Autodesk Fusion 360 part; units mm, degrees
note: some values were not read from the file. Set by a fixed rule: which sketch regions a step uses.
(part 2 of 2)
sketch "Sketch46" plane through (0, 0, 3) normal (0, 0, 1) x (-1, 0, 0)
  line L0 (110.0265, 86.5) -> (110.0265, 76.5)
  line L1 (110.0265, 76.5) -> (120.0265, 76.5)
  line L2 (120.0265, 76.5) -> (120.0265, 5)
  line L3 (116.5265, 5) -> (116.5265, 73)
  line L4 (116.5265, 73) -> (106.5265, 73)
  line L5 (106.5265, 73) -> (106.5265, 83)
  line L6 (106.5265, 83) -> (-17.7235, 83)
  line L7 (-21.2235, 86.5) -> (110.0265, 86.5)
  line L8 (-34.7235, -90) -> (123.5265, -90)
  line L9 (123.5265, -90) -> (123.5265, 90)
  line L10 (123.5265, 90) -> (-34.7235, 90)
  line L11 (-34.7235, 90) -> (-34.7235, -90)
  line L12 (12.9015, 40) -> (12.9015, 81)
  line L13 (75.9015, 81) -> (75.9015, 40)
  line L14 (75.9015, 40) -> (12.9015, 40)
  circle A0 centre (59.4015, -45) radius 2.5
  circle A1 centre (59.4015, 15) radius 2.5
  circle A2 centre (59.4015, -15) radius 2.5
  circle A3 centre (78.4015, -45) radius 2.5
  circle A4 centre (78.4015, -15) radius 2.5
  line L15 (-5.7917, -72.9167) -> (-5.7917, -61.9167)
  line L16 (-5.7917, -61.9167) -> (22.9083, -61.9167)
  line L17 (22.9083, -61.9167) -> (22.9083, -72.9167)
  line L18 (22.9083, -72.9167) -> (-5.7917, -72.9167)
  line L19 (-17.7235, -83.5) -> (106.5265, -83.5)
  line L20 (106.5265, -83.5) -> (106.5265, -73)
  line L21 (106.5265, -73) -> (116.5265, -73)
  line L22 (116.5265, -73) -> (116.5265, 0)
  line L23 (116.5265, 0) -> (120.0265, 0)
  line L24 (120.0265, 0) -> (120.0265, -76.5)
  line L25 (120.0265, -76.5) -> (110.0265, -76.5)
  line L26 (110.0265, -76.5) -> (110.0265, -87)
  line L27 (110.0265, -87) -> (-21.2235, -87)
  line L28 (-21.2235, -87) -> (-21.2235, -76.5)
  line L29 (-21.2235, -76.5) -> (-31.2235, -76.5)
  line L30 (-31.2235, -76.5) -> (-31.2235, 0)
  line L31 (-31.2235, 0) -> (-27.7235, 0)
  line L32 (-27.7235, 0) -> (-27.7235, -73)
  line L33 (-27.7235, -73) -> (-17.7235, -73)
  line L34 (-17.7235, -73) -> (-17.7235, -83.5)
  circle A5 centre (116.7765, 83.25) radius 2.5
  line L35 (12.9015, 81) -> (75.9015, 81)
  circle A6 centre (78.4015, 15) radius 2.5
  line L36 (-27.7235, 5) -> (-31.2235, 5)
  line L37 (-31.2235, 5) -> (-31.2235, 76.5)
  line L38 (-31.2235, 76.5) -> (-21.2235, 76.5)
  line L39 (-21.2235, 76.5) -> (-21.2235, 86.5)
  line L40 (-17.7235, 83) -> (-17.7235, 73)
  line L41 (-17.7235, 73) -> (-27.7235, 73)
  line L42 (-27.7235, 73) -> (-27.7235, 5)
  circle A7 centre (-27.9735, 83.25) radius 2.5
  circle A8 centre (10.4015, -15) radius 2.5
  circle A9 centre (10.4015, 15) radius 2.5
  circle A10 centre (29.4015, -45) radius 2.5
  circle A11 centre (29.4015, -15) radius 2.5
  circle A12 centre (29.4015, 15) radius 2.5
  circle A13 centre (10.4015, -45) radius 2.5
  circle A14 centre (-4.7235, 40) radius 3.5
  line L43 (120.0265, 5) -> (116.5265, 5)
  dimension "d201" = 5
  dimension "d350" = 6.75
  measures "d201" diameter of A5
  measures "d350" distance of L10 A5.centre
extrude "Extrude43" cut sketch "Sketch46" against normal blind 3 contours A5 bodies 2
sketch "Sketch47" plane through (0, 0, 3) normal (0, 0, 1) x (-1, 0, 0)
  line L0 (-17.7235, -83.5) -> (106.5265, -83.5)
  line L1 (106.5265, -83.5) -> (106.5265, -73)
  line L2 (106.5265, -73) -> (116.5265, -73)
  line L3 (116.5265, -73) -> (116.5265, 0)
  line L4 (116.5265, 0) -> (120.0265, 0)
  line L5 (120.0265, 0) -> (120.0265, -76.5)
  line L6 (120.0265, -76.5) -> (110.0265, -76.5)
  line L7 (110.0265, -76.5) -> (110.0265, -87)
  line L8 (110.0265, -87) -> (-21.2235, -87)
  line L9 (-21.2235, -87) -> (-21.2235, -76.5)
  line L10 (-21.2235, -76.5) -> (-31.2235, -76.5)
  line L11 (-31.2235, -76.5) -> (-31.2235, 0)
  line L12 (-31.2235, 0) -> (-27.7235, 0)
  line L13 (-27.7235, 0) -> (-27.7235, -73)
  line L14 (-27.7235, -73) -> (-17.7235, -73)
  line L15 (-17.7235, -73) -> (-17.7235, -83.5)
  line L16 (-5.7917, -72.9167) -> (-5.7917, -61.9167)
  line L17 (-5.7917, -61.9167) -> (22.9083, -61.9167)
  line L18 (22.9083, -61.9167) -> (22.9083, -72.9167)
  line L19 (22.9083, -72.9167) -> (-5.7917, -72.9167)
  circle A0 centre (78.4015, -15) radius 2.5
  circle A1 centre (78.4015, -45) radius 2.5
  circle A2 centre (59.4015, -15) radius 2.5
  circle A3 centre (59.4015, 15) radius 2.5
  circle A4 centre (59.4015, -45) radius 2.5
  line L20 (12.9015, 40) -> (12.9015, 81)
  line L21 (12.9015, 81) -> (75.9015, 81)
  line L22 (75.9015, 81) -> (75.9015, 40)
  line L23 (75.9015, 40) -> (12.9015, 40)
  line L24 (-34.7235, -90) -> (123.5265, -90)
  line L25 (123.5265, -90) -> (123.5265, 90)
  line L26 (123.5265, 90) -> (-34.7235, 90)
  line L27 (-34.7235, 90) -> (-34.7235, -90)
  line L28 (110.0265, 86.5) -> (110.0265, 76.5)
  line L29 (110.0265, 76.5) -> (120.0265, 76.5)
  line L30 (120.0265, 76.5) -> (120.0265, 5)
  line L31 (116.5265, 5) -> (116.5265, 73)
  line L32 (116.5265, 73) -> (106.5265, 73)
  line L33 (106.5265, 73) -> (106.5265, 83)
  line L34 (-21.2235, 86.5) -> (110.0265, 86.5)
  line L35 (110.0265, -87) -> (110.0265, -76.5)
  circle A5 centre (116.7765, -83.25) radius 2.5
  line L36 (106.5265, 83) -> (-17.7235, 83)
  circle A6 centre (78.4015, 15) radius 2.5
  line L37 (-17.7235, 83) -> (-17.7235, 73)
  line L38 (-17.7235, 73) -> (-27.7235, 73)
  line L39 (-27.7235, 73) -> (-27.7235, 5)
  line L40 (-27.7235, 5) -> (-31.2235, 5)
  line L41 (-31.2235, 5) -> (-31.2235, 76.5)
  line L42 (-31.2235, 76.5) -> (-21.2235, 76.5)
  line L43 (-21.2235, 76.5) -> (-21.2235, 86.5)
  circle A7 centre (-27.9735, 83.25) radius 2.5
  circle A8 centre (116.7765, 83.25) radius 2.5
  circle A9 centre (10.4015, -45) radius 2.5
  circle A10 centre (29.4015, 15) radius 2.5
  circle A11 centre (29.4015, -15) radius 2.5
  circle A12 centre (29.4015, -45) radius 2.5
  circle A13 centre (10.4015, 15) radius 2.5
  circle A14 centre (10.4015, -15) radius 2.5
  circle A15 centre (-4.7235, 40) radius 3.5
  line L44 (120.0265, 5) -> (116.5265, 5)
  dimension "d204" = 5
  dimension "d351" = 6.75
  constraint coincident L6.end L7.start
  measures "d204" diameter of A5
  measures "d351" distance of L24 A5.centre
extrude "Extrude44" cut sketch "Sketch47" against normal blind 3 contours A5 bodies 2
sketch "Sketch48" plane through (0, 0, 3) normal (0, 0, 1) x (-1, 0, 0)
  line L0 (110.0265, 86.5) -> (110.0265, 76.5)
  line L1 (110.0265, 76.5) -> (120.0265, 76.5)
  line L2 (120.0265, 76.5) -> (120.0265, 5)
  line L3 (116.5265, 5) -> (116.5265, 73)
  line L4 (116.5265, 73) -> (106.5265, 73)
  line L5 (106.5265, 73) -> (106.5265, 83)
  line L6 (106.5265, 83) -> (-17.7235, 83)
  line L7 (-21.2235, 86.5) -> (110.0265, 86.5)
  line L8 (-34.7235, -90) -> (123.5265, -90)
  line L9 (123.5265, -90) -> (123.5265, 90)
  line L10 (123.5265, 90) -> (-34.7235, 90)
  line L11 (-34.7235, 90) -> (-34.7235, -90)
  line L12 (12.9015, 40) -> (12.9015, 81)
  line L13 (75.9015, 81) -> (75.9015, 40)
  line L14 (75.9015, 40) -> (12.9015, 40)
  circle A0 centre (59.4015, -45) radius 2.5
  circle A1 centre (59.4015, 15) radius 2.5
  circle A2 centre (59.4015, -15) radius 2.5
  circle A3 centre (78.4015, -45) radius 2.5
  circle A4 centre (78.4015, -15) radius 2.5
  line L15 (-5.7917, -72.9167) -> (-5.7917, -61.9167)
  line L16 (-5.7917, -61.9167) -> (22.9083, -61.9167)
  line L17 (22.9083, -61.9167) -> (22.9083, -72.9167)
  line L18 (22.9083, -72.9167) -> (-5.7917, -72.9167)
  line L19 (-17.7235, -83.5) -> (106.5265, -83.5)
  line L20 (106.5265, -83.5) -> (106.5265, -73)
  line L21 (106.5265, -73) -> (116.5265, -73)
  line L22 (116.5265, -73) -> (116.5265, 0)
  line L23 (116.5265, 0) -> (120.0265, 0)
  line L24 (120.0265, 0) -> (120.0265, -76.5)
  line L25 (120.0265, -76.5) -> (110.0265, -76.5)
  line L26 (110.0265, -76.5) -> (110.0265, -87)
  line L27 (110.0265, -87) -> (-21.2235, -87)
  line L28 (-21.2235, -87) -> (-21.2235, -76.5)
  line L29 (-21.2235, -76.5) -> (-31.2235, -76.5)
  line L30 (-31.2235, -76.5) -> (-31.2235, 0)
  line L31 (-31.2235, 0) -> (-27.7235, 0)
  line L32 (-27.7235, 0) -> (-27.7235, -73)
  line L33 (-27.7235, -73) -> (-17.7235, -73)
  line L34 (-17.7235, -73) -> (-17.7235, -83.5)
  circle A5 centre (-27.9735, -83.25) radius 2.5
  line L35 (12.9015, 81) -> (75.9015, 81)
  circle A6 centre (78.4015, 15) radius 2.5
  line L36 (-17.7235, 83) -> (-17.7235, 73)
  line L37 (-17.7235, 73) -> (-27.7235, 73)
  line L38 (-27.7235, 73) -> (-27.7235, 5)
  line L39 (-27.7235, 5) -> (-31.2235, 5)
  line L40 (-31.2235, 5) -> (-31.2235, 76.5)
  line L41 (-31.2235, 76.5) -> (-21.2235, 76.5)
  line L42 (-21.2235, 76.5) -> (-21.2235, 86.5)
  circle A7 centre (-27.9735, 83.25) radius 2.5
  circle A8 centre (116.7765, 83.25) radius 2.5
  circle A9 centre (116.7765, -83.25) radius 2.5
  circle A10 centre (10.4015, -15) radius 2.5
  circle A11 centre (10.4015, 15) radius 2.5
  circle A12 centre (29.4015, -45) radius 2.5
  circle A13 centre (29.4015, -15) radius 2.5
  circle A14 centre (29.4015, 15) radius 2.5
  circle A15 centre (10.4015, -45) radius 2.5
  circle A16 centre (-4.7235, 40) radius 3.5
  line L43 (120.0265, 5) -> (116.5265, 5)
  dimension "d207" = 5
  dimension "d352" = 6.75
  measures "d207" diameter of A5
  measures "d352" distance of L8 A5.centre
extrude "Extrude45" cut sketch "Sketch48" against normal blind 3 contours A5 bodies 2
move_body "Move11" bodies 2 to x (1, 0, 0) y (0, 1, 0) z (0, 0, 1) at (274.2168, 184.9353, 0)
sketch "Sketch71" plane through (0, 0, 3) normal (0, 0, 1) x (-1, 0, 0)
  circle A0 centre (-157.4403, -268.1853) radius 2.5
  circle A1 centre (-302.1903, -101.6853) radius 2.5
  line L0 (-291.9403, -268.4353) -> (-167.6903, -268.4353)
  line L1 (-167.6903, -268.4353) -> (-167.6903, -257.9353)
  line L2 (-167.6903, -257.9353) -> (-157.6903, -257.9353)
  line L3 (-157.6903, -257.9353) -> (-157.6903, -184.9353)
  line L4 (-157.6903, -184.9353) -> (-154.1903, -184.9353)
  line L5 (-154.1903, -184.9353) -> (-154.1903, -261.4353)
  line L6 (-154.1903, -261.4353) -> (-164.1903, -261.4353)
  line L7 (-164.1903, -261.4353) -> (-164.1903, -271.9353)
  line L8 (-164.1903, -271.9353) -> (-295.4403, -271.9353)
  line L9 (-295.4403, -271.9353) -> (-295.4403, -261.4353)
  line L10 (-295.4403, -261.4353) -> (-305.4403, -261.4353)
  line L11 (-305.4403, -261.4353) -> (-305.4403, -184.9353)
  line L12 (-305.4403, -184.9353) -> (-301.9403, -184.9353)
  line L13 (-301.9403, -184.9353) -> (-301.9403, -257.9353)
  line L14 (-301.9403, -257.9353) -> (-291.9403, -257.9353)
  line L15 (-291.9403, -257.9353) -> (-291.9403, -268.4353)
  circle A2 centre (-278.9403, -144.9353) radius 3.5
  line L16 (-308.9403, -274.9353) -> (-150.6903, -274.9353)
  line L17 (-150.6903, -274.9353) -> (-150.6903, -94.9353)
  line L18 (-150.6903, -94.9353) -> (-308.9403, -94.9353)
  line L19 (-308.9403, -94.9353) -> (-308.9403, -274.9353)
  line L20 (-261.3153, -144.9353) -> (-261.3153, -103.9353)
  line L21 (-261.3153, -103.9353) -> (-198.3153, -103.9353)
  line L22 (-198.3153, -103.9353) -> (-198.3153, -144.9353)
  line L23 (-198.3153, -144.9353) -> (-261.3153, -144.9353)
  circle A3 centre (-263.8153, -229.9353) radius 2.5
  circle A4 centre (-244.8153, -169.9353) radius 2.5
  circle A5 centre (-195.8153, -199.9353) radius 2.5
  circle A6 centre (-195.8153, -169.9353) radius 2.5
  circle A7 centre (-195.8153, -229.9353) radius 2.5
  circle A8 centre (-244.8153, -199.9353) radius 2.5
  circle A9 centre (-244.8153, -229.9353) radius 2.5
  circle A10 centre (-263.8153, -169.9353) radius 2.5
  circle A11 centre (-214.8153, -199.9353) radius 2.5
  circle A12 centre (-214.8153, -169.9353) radius 2.5
  circle A13 centre (-214.8153, -229.9353) radius 2.5
  circle A14 centre (-263.8153, -199.9353) radius 2.5
  line L24 (-280.0085, -257.8521) -> (-280.0085, -246.8521)
  line L25 (-280.0085, -246.8521) -> (-251.3085, -246.8521)
  line L26 (-251.3085, -246.8521) -> (-251.3085, -257.8521)
  line L27 (-251.3085, -257.8521) -> (-280.0085, -257.8521)
  line L28 (-301.9403, -111.9353) -> (-301.9403, -179.9353)
  line L29 (-301.9403, -179.9353) -> (-305.4403, -179.9353)
  line L30 (-305.4403, -179.9353) -> (-305.4403, -108.4353)
  line L31 (-305.4403, -108.4353) -> (-295.4403, -108.4353)
  line L32 (-295.4403, -108.4353) -> (-295.4403, -98.4353)
  line L33 (-295.4403, -98.4353) -> (-164.1903, -98.4353)
  line L34 (-164.1903, -98.4353) -> (-164.1903, -108.4353)
  line L35 (-164.1903, -108.4353) -> (-154.1903, -108.4353)
  line L36 (-154.1903, -108.4353) -> (-154.1903, -179.9353)
  line L37 (-157.6903, -179.9353) -> (-157.6903, -111.9353)
  line L38 (-157.6903, -111.9353) -> (-167.6903, -111.9353)
  line L39 (-167.6903, -111.9353) -> (-167.6903, -101.9353)
  line L40 (-167.6903, -101.9353) -> (-291.9403, -101.9353)
  line L41 (-291.9403, -101.9353) -> (-291.9403, -111.9353)
  line L42 (-291.9403, -111.9353) -> (-301.9403, -111.9353)
  circle A15 centre (-157.4403, -101.6853) radius 2.5
  circle A16 centre (-302.1903, -268.1853) radius 2.5
  line L43 (-208.2528, -247.9239) -> (-194.7528, -247.9239)
  line L44 (-194.7528, -247.9239) -> (-194.7528, -254.4239)
  line L45 (-194.7528, -254.4239) -> (-208.2528, -254.4239)
  line L46 (-208.2528, -254.4239) -> (-208.2528, -247.9239)
  line L47 (-154.1903, -179.9353) -> (-157.6903, -179.9353)
  dimension "d370" = 13.5
  dimension "d371" = 6.5
  constraint horizontal L43
  constraint vertical L44
  constraint horizontal L45
  constraint vertical L46
  measures "d370" distance of L43.start L43.end
  measures "d371" distance of L43 L45
extrude "Extrude74" cut sketch "Sketch71" against normal blind 3 contours L43 L44 L45 L46 bodies 2
sketch "Sketch72" plane through (0, 0, 3) normal (0, 0, 1) x (-1, 0, 0)
  circle A0 centre (-302.1903, -268.1853) radius 2.5
  circle A1 centre (-157.4403, -101.6853) radius 2.5
  line L0 (-301.9403, -111.9353) -> (-301.9403, -179.9353)
  line L1 (-301.9403, -179.9353) -> (-305.4403, -179.9353)
  line L2 (-305.4403, -179.9353) -> (-305.4403, -108.4353)
  line L3 (-305.4403, -108.4353) -> (-295.4403, -108.4353)
  line L4 (-295.4403, -108.4353) -> (-295.4403, -98.4353)
  line L5 (-295.4403, -98.4353) -> (-164.1903, -98.4353)
  line L6 (-164.1903, -98.4353) -> (-164.1903, -108.4353)
  line L7 (-164.1903, -108.4353) -> (-154.1903, -108.4353)
  line L8 (-154.1903, -108.4353) -> (-154.1903, -179.9353)
  line L9 (-157.6903, -179.9353) -> (-157.6903, -111.9353)
  line L10 (-157.6903, -111.9353) -> (-167.6903, -111.9353)
  line L11 (-167.6903, -111.9353) -> (-167.6903, -101.9353)
  line L12 (-167.6903, -101.9353) -> (-291.9403, -101.9353)
  line L13 (-291.9403, -101.9353) -> (-291.9403, -111.9353)
  line L14 (-291.9403, -111.9353) -> (-301.9403, -111.9353)
  line L15 (-280.0085, -257.8521) -> (-280.0085, -246.8521)
  line L16 (-280.0085, -246.8521) -> (-251.3085, -246.8521)
  line L17 (-251.3085, -246.8521) -> (-251.3085, -257.8521)
  line L18 (-251.3085, -257.8521) -> (-280.0085, -257.8521)
  circle A2 centre (-263.8153, -199.9353) radius 2.5
  circle A3 centre (-214.8153, -229.9353) radius 2.5
  circle A4 centre (-214.8153, -169.9353) radius 2.5
  circle A5 centre (-214.8153, -199.9353) radius 2.5
  circle A6 centre (-263.8153, -169.9353) radius 2.5
  circle A7 centre (-244.8153, -229.9353) radius 2.5
  circle A8 centre (-244.8153, -199.9353) radius 2.5
  circle A9 centre (-195.8153, -229.9353) radius 2.5
  circle A10 centre (-195.8153, -169.9353) radius 2.5
  circle A11 centre (-195.8153, -199.9353) radius 2.5
  circle A12 centre (-244.8153, -169.9353) radius 2.5
  circle A13 centre (-263.8153, -229.9353) radius 2.5
  line L19 (-261.3153, -144.9353) -> (-261.3153, -103.9353)
  line L20 (-261.3153, -103.9353) -> (-198.3153, -103.9353)
  line L21 (-198.3153, -103.9353) -> (-198.3153, -144.9353)
  line L22 (-198.3153, -144.9353) -> (-261.3153, -144.9353)
  line L23 (-308.9403, -274.9353) -> (-150.6903, -274.9353)
  line L24 (-150.6903, -274.9353) -> (-150.6903, -94.9353)
  line L25 (-150.6903, -94.9353) -> (-308.9403, -94.9353)
  line L26 (-308.9403, -94.9353) -> (-308.9403, -274.9353)
  circle A14 centre (-278.9403, -144.9353) radius 3.5
  line L27 (-291.9403, -268.4353) -> (-167.6903, -268.4353)
  line L28 (-167.6903, -268.4353) -> (-167.6903, -257.9353)
  line L29 (-167.6903, -257.9353) -> (-157.6903, -257.9353)
  line L30 (-157.6903, -257.9353) -> (-157.6903, -184.9353)
  line L31 (-157.6903, -184.9353) -> (-154.1903, -184.9353)
  line L32 (-154.1903, -184.9353) -> (-154.1903, -261.4353)
  line L33 (-154.1903, -261.4353) -> (-164.1903, -261.4353)
  line L34 (-164.1903, -261.4353) -> (-164.1903, -271.9353)
  line L35 (-164.1903, -271.9353) -> (-295.4403, -271.9353)
  line L36 (-295.4403, -271.9353) -> (-295.4403, -261.4353)
  line L37 (-295.4403, -261.4353) -> (-305.4403, -261.4353)
  line L38 (-305.4403, -261.4353) -> (-305.4403, -184.9353)
  line L39 (-305.4403, -184.9353) -> (-301.9403, -184.9353)
  line L40 (-301.9403, -184.9353) -> (-301.9403, -257.9353)
  line L41 (-301.9403, -257.9353) -> (-291.9403, -257.9353)
  line L42 (-291.9403, -257.9353) -> (-291.9403, -268.4353)
  circle A15 centre (-302.1903, -101.6853) radius 2.5
  circle A16 centre (-157.4403, -268.1853) radius 2.5
  line L43 (-194.7528, -247.9239) -> (-194.7528, -254.4239)
  line L44 (-194.7528, -254.4239) -> (-208.2528, -254.4239)
  line L45 (-208.2528, -254.4239) -> (-208.2528, -247.9239)
  line L46 (-208.2528, -247.9239) -> (-194.7528, -247.9239)
  line L47 (-208.2528, -254.4239) -> (-208.2528, -256.9239)
  line L48 (-208.2528, -256.9239) -> (-194.7528, -256.9239)
  line L49 (-194.7528, -256.9239) -> (-194.7528, -254.4239)
  line L50 (-154.1903, -179.9353) -> (-157.6903, -179.9353)
  dimension "d374" = 2.5
  constraint coincident L44.end L45.start
  constraint perpendicular L44 L47
  constraint perpendicular L47 L48
  constraint coincident L43.end L44.start
  constraint perpendicular L44 L49
  measures "d374" distance of L44 L48
extrude "Extrude75" add sketch "Sketch72" along normal blind 10 contours L44 L47 L48 L49 bodies 2
sketch "Sketch73" plane through (0, 254.4239, 0) normal (0, -1, 0) x (1, 0, 0)
  line L0 (194.7528, 3) -> (194.7528, 0)
  line L1 (194.7528, 0) -> (208.2528, 0)
  line L2 (208.2528, 0) -> (208.2528, 3)
  line L3 (208.2528, 3) -> (208.2528, 13)
  line L4 (208.2528, 13) -> (194.7528, 13)
  line L5 (194.7528, 13) -> (194.7528, 3)
  line L6 (208.2528, 13) -> (194.7528, 13)
  line L7 (194.7528, 13) -> (194.7528, 11)
  line L8 (194.7528, 11) -> (208.2528, 11)
  line L9 (208.2528, 11) -> (208.2528, 13)
  dimension "d380" = 2
  constraint horizontal L6
  constraint vertical L7
  constraint horizontal L8
  constraint vertical L9
  constraint coincident L3.end L4.start
  measures "d380" distance of L3.end L8.end
extrude "Extrude76" add sketch "Sketch73" along normal blind 6.5 contours L3 L4 L5 L6 L7 L8 L9 bodies 2
sketch "Sketch74" plane through (0, -122.0134, 0) normal (0, -1, 0) x (1, 0, 0)
  line L0 (156.0637, 0) -> (314.3137, 0)
  line L1 (314.3137, 0) -> (314.3137, 225)
  line L2 (314.3137, 225) -> (156.0637, 225)
  line L3 (156.0637, 225) -> (156.0637, 0)
  circle A0 centre (247.3137, 13) radius 1.8
  circle A1 centre (247.3137, 37) radius 1.8
  circle A2 centre (271.3137, 37) radius 1.8
  circle A3 centre (271.3137, 13) radius 1.8
  circle A4 centre (259.3137, 25) radius 14
  circle A5 centre (199.0637, 37) radius 1.8
  circle A6 centre (223.0637, 37) radius 1.8
  circle A7 centre (199.0637, 13) radius 1.8
  circle A8 centre (223.0637, 13) radius 1.8
  circle A9 centre (211.0637, 25) radius 14
  dimension "d391" = 3.6
  dimension "d392" = 3.6
  dimension "d393" = 3.6
  dimension "d394" = 3.6
  dimension "d395" = 24
  dimension "d398" = 28
  dimension "d399" = 3.6
  dimension "d400" = 3.6
  dimension "d401" = 3.6
  dimension "d402" = 3.6
  dimension "d403" = 24
  dimension "d406" = 28
  measures "d391" diameter of A0
  measures "d392" diameter of A1
  measures "d393" diameter of A2
  measures "d394" diameter of A3
  measures "d395" horizontal distance of A1.centre A2.centre
  measures "d398" diameter of A4
  measures "d399" diameter of A5
  measures "d400" diameter of A6
  measures "d401" diameter of A7
  measures "d402" diameter of A8
  measures "d403" distance of A5.centre A6.centre
  measures "d406" diameter of A9
extrude "Extrude77" cut sketch "Sketch74" against normal blind 5 contours A0 | A1 | A2 | A3 | A4 | A5 | A6 | A7 | A8 | A9 bodies 1
sketch "Sketch77" plane through (154.1903, 0, 0) normal (-1, 0, 0) x (0, -1, 0)
  line L0 (-261.4353, 3) -> (-184.9353, 3)
  line L1 (-184.9353, 3) -> (-184.9353, 83)
  line L2 (-184.9353, 83) -> (-261.4353, 83)
  line L3 (-261.4353, 83) -> (-261.4353, 3)
  line L4 (-254.4835, 79.5) -> (-191.8871, 79.5)
  line L5 (-188.4353, 75.8743) -> (-188.4353, 10.1257)
  line L6 (-191.8871, 6.5) -> (-254.4835, 6.5)
  line L7 (-257.9353, 10.1257) -> (-257.9353, 75.8743)
  line L8 (-226.6371, 43) -> (-257.9353, 75.8743)
  line L9 (-219.7335, 43) -> (-188.4353, 75.8743)
  line L10 (-191.8871, 79.5) -> (-223.1853, 46.6257)
  line L11 (-254.4835, 79.5) -> (-223.1853, 46.6257)
  line L12 (-254.4835, 6.5) -> (-223.1853, 39.3743)
  line L13 (-226.6371, 43) -> (-257.9353, 10.1257)
  line L14 (-188.4353, 10.1257) -> (-219.7335, 43)
  line L15 (-223.1853, 39.3743) -> (-191.8871, 6.5)
  dimension "d445" = 3.5
  dimension "d446" = 3.5
  dimension "d447" = 3.5
  dimension "d448" = 3.5
  constraint horizontal L4
  constraint vertical L5
  constraint horizontal L6
  constraint vertical L7
  constraint parallel L9 L10
  measures "d445" distance of L2 L4
  measures "d446" distance of L1 L5
  measures "d447" distance of L3 L7
  measures "d448" distance of L0 L6
extrude "Extrude81" cut sketch "Sketch77" against normal blind 5 contours L4 L10 L11 | L5 L9 L14 | L6 L12 L15 | L7 L8 L13 bodies 2
sketch "Sketch78" plane through (305.4403, 0, 0) normal (1, 0, 0) x (0, 1, 0)
  line L0 (184.9353, 3) -> (261.4353, 3)
  line L1 (261.4353, 3) -> (261.4353, 83)
  line L2 (261.4353, 83) -> (184.9353, 83)
  line L3 (184.9353, 83) -> (184.9353, 3)
  line L4 (191.8871, 79.5) -> (254.4835, 79.5)
  line L5 (257.9353, 75.8743) -> (257.9353, 10.1257)
  line L6 (254.4835, 6.5) -> (191.8871, 6.5)
  line L7 (188.4353, 10.1257) -> (188.4353, 75.8743)
  line L8 (219.7335, 43) -> (188.4353, 75.8743)
  line L9 (223.1853, 39.3743) -> (254.4835, 6.5)
  line L10 (226.6371, 43) -> (257.9353, 75.8743)
  line L11 (254.4835, 79.5) -> (223.1853, 46.6257)
  line L12 (191.8871, 79.5) -> (223.1853, 46.6257)
  line L13 (257.9353, 10.1257) -> (226.6371, 43)
  line L14 (219.7335, 43) -> (188.4353, 10.1257)
  line L15 (191.8871, 6.5) -> (223.1853, 39.3743)
  dimension "d453" = 3.5
  dimension "d454" = 3.5
  dimension "d455" = 3.5
  dimension "d456" = 3.5
  constraint horizontal L4
  constraint vertical L5
  constraint horizontal L6
  constraint vertical L7
  constraint parallel L10 L11
  constraint parallel L14 L15
  measures "d453" distance of L2 L4
  measures "d454" distance of L0 L6
  measures "d455" distance of L1 L5
  measures "d456" distance of L3 L7
extrude "Extrude82" cut sketch "Sketch78" against normal blind 5 contours L4 L11 L12 | L5 L10 L13 | L6 L9 L15 | L7 L8 L14 bodies 2
